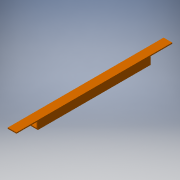
# Autodesk Inventor part: 2018 Cube Back Stop Top_Botom
Saved by Autodesk Inventor 2018 (Build 220112000, 112)
## iProperties
Created: 2018-01-23
Part Number: 2018 Cube Back Stop Top_Botom
Material: Generic
Document SubType Name: Modeling
Designer: Apple
Density: 1 g/cm^3
Appearance: Default
Author: Apple
Autodesk Inventor part; units mm, degrees
ref_plane "YZ Plane" through (0, 0, 0) normal (1, 0, 0) x (0, 1, 0)
ref_plane "XZ Plane" through (0, 0, 0) normal (0, 1, 0) x (-1, 0, 0)
ref_plane "XY Plane" through (0, 0, 0) normal (0, 0, 1) x (1, 0, 0)
sketch "Sketch1" plane through (0, 0, 0) normal (0, 0, 1) x (1, 0, 0)
  line L0 (190.5, 3.175) -> (0, 3.175) projected
  line L1 (25.0046, 3.175) -> (50.4046, 3.175)
  line L2 (50.4046, 3.175) -> (50.4046, -22.225)
  line L3 (50.4046, -22.225) -> (25.0046, -22.225)
  line L4 (25.0046, -22.225) -> (25.0046, 3.175)
  line L5 (28.1796, 0) -> (47.2296, 0)
  line L6 (47.2296, 0) -> (47.2296, -19.05)
  line L7 (47.2296, -19.05) -> (28.1796, -19.05)
  line L8 (28.1796, -19.05) -> (28.1796, 0)
  point P0 (0, 0)
  dimension "d0" = 25.4
  dimension "d1" = 25.4
  dimension "d2" = 3.175
  constraints: 16 end point, 4 parallel, 2 perpendicular, 1 horizontal, 1 point on line, 3 other
  measures "d0" distance of L3.end L1.start
  measures "d1" distance of L2.end L3.end
  measures "d2" distance between parallel lines of L4 L8
ref_plane "Work Plane1" through (0, 0, -461.1116) normal (0, 0, -1) x (0, 1, 0)
extrude "Extrusion1" add sketch "Sketch1" against normal up to surface (461.1116 mm away)
sketch "Sketch2" plane through (50.4046, -22.225, 0) normal (1, 0, 0) x (0, 0, -1)
  line L0 (461.1116, 0) -> (461.1116, 25.4) projected
  line L1 (0, 25.4) -> (461.1116, 25.4) projected
  line L2 (0, 25.4) -> (0, 0) projected
  line L3 (0, 0) -> (461.1116, 0) projected
  line L4 (0, 0) -> (63.5, 0)
  line L5 (63.5, 0) -> (63.5, 22.225)
  line L6 (63.5, 22.225) -> (0, 22.225)
  line L7 (0, 22.225) -> (0, 0)
  line L8 (461.1116, 0) -> (397.6116, 0)
  line L9 (397.6116, 0) -> (397.6116, 22.225)
  line L10 (397.6116, 22.225) -> (461.1116, 22.225)
  line L11 (461.1116, 22.225) -> (461.1116, 0)
  point P0 (0, 22.225)
  dimension "d5" = 63.5
  dimension "d6" = 22.225
  dimension "d7" = 63.5
  dimension "d8" = 22.225
  constraints: 16 end point, 4 parallel, 2 horizontal, 2 perpendicular
  measures "d5" distance of L5.end L6.end
  measures "d6" distance of L4.end L5.end
  measures "d7" distance of L9.end L10.end
  measures "d8" distance of L8.end L9.end
extrude "Extrusion2" cut sketch "Sketch2" against normal through all contours L3 L9 L10 L0 | L3 L2 L6 L5
equation "\"d7\" = d5"
equation "\"d8\" = d6"
body "Solid1"
